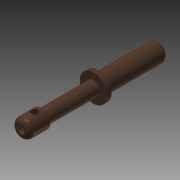
# Autodesk Inventor part: ConnectorPin
Saved by Autodesk Inventor 2014 SP2 (Build 180246200, 246)
## iProperties
Created: 2015-09-20
Part Number: ConnectorPin
Material: Generic
Document SubType Name: Modeling
Designer: Lukasz Szmit
Density: 1 g/cm^3
Appearance: Default
Mass: 0.322592 g
Surface Area: 4.28963 cm^2
Volume: 0.322592 cm^3
Author: Lukasz Szmit
Autodesk Inventor part; units mm, degrees
ref_plane "YZ Plane" through (0, 0, 0) normal (1, 0, 0) x (0, 1, 0)
ref_plane "XZ Plane" through (0, 0, 0) normal (0, 1, 0) x (-1, 0, 0)
sketch "Sketch1" plane through (0, 0, 0) normal (0, 0, 1) x (1, 0, 0)
  line L0 (-16.5001, 0.5) -> (-16.5001, -0.5)
  line L1 (-13.5001, 14) -> (-13.5001, -15.5)
  line L2 (-15.5001, 0.5) -> (-16.5001, 0.5)
  line L3 (-15.5001, 0.5) -> (-15.5001, 13)
  arc A0 (-14.5001, 14) -> (-15.5001, 13) centre (-14.5001, 13) ccw
  line L4 (-14.5001, 14) -> (-13.5001, 14)
  line L5 (-16.5001, -0.5) -> (-15.0001, -0.5)
  line L6 (-15.0001, -12) -> (-15.0001, -0.5)
  line L7 (-15.5001, -12) -> (-15.0001, -12)
  line L8 (-15.5001, -15.5318) -> (-15.5001, -12)
  line L9 (-13.5001, -15.5) -> (-14.2501, -15.5)
  arc A1 (-15.5001, -15.5318) -> (-14.2501, -16.5) centre (-14.5001, -15.5318) ccw
  line L10 (-14.2501, -15.5) -> (-14.2501, -16.5)
  dimension "d3" = 0.75
  dimension "d10" = 30.5
  dimension "d11" = 1
  dimension "d12" = 2
  dimension "d13" = 1
  dimension "d14" = 1.5
  dimension "d15" = 1
  dimension "d16" = 1.5
  dimension "d17" = 1
  dimension "d18" = 0.5
  dimension "d19" = 4.5
  dimension "d20" = 14.5
  dimension "d22" = 11.5
  dimension "d23" = 2
  dimension "d24" = 1
  constraints: 22 end point, 4 point on circle, 3 perpendicular, 3 tangent, 2 centre point, 2 parallel, 1 equal radius
  measures "d3" distance of L1.end L9.end
  measures "d10" vertical distance of L10.end L1.start
  measures "d11" distance of L0.start L0.end
  measures "d12" distance between parallel lines of L3 L1
  measures "d13" radius of A0
  measures "d14" distance between parallel lines of L6 L1
  measures "d15" distance of L2.start L0.start
  measures "d16" distance of L0.end L5.end
  measures "d17" radius of A1
  measures "d18" distance of L7.start L6.start
  measures "d19" vertical distance of L10.end L7.start
  measures "d20" vertical distance of L5.end L1.start
  measures "d22" distance of L6.start L5.end
  measures "d23" distance between parallel lines of L1 L8
  measures "d24" distance of L9.end L10.end
revolve "Revolution1" add sketch "Sketch1" angle 360 about axis through (-13.5001, 14, 0) along (0, -1, 0)
ref_plane "Work Plane1" through (-13.5001, -13.7659, 2) normal (0, 0, 1) x (1, 0, 0)
sketch "Sketch2" plane through (-13.5001, -13.7659, 2) normal (0, 0, 1) x (1, 0, 0)
  line L0 (0, -1.7659) -> (0, 1.7659) construction
  line L1 (2.2361, 13.2659) -> (-2.2361, 13.2659) construction
  line L2 (-2.2361, 13.2659) -> (-2.2361, 14.2659) construction
  line L3 (-2.2361, 14.2659) -> (0, 14.2659) construction
  line L4 (0, 14.2659) -> (0, 26.7659) construction
  line L5 (2.2361, 14.2659) -> (2.2361, 13.2659) construction
  line L6 (0, 14.2659) -> (2.2361, 14.2659) construction
  point P0 (13.5001, 13.7659)
  point P1 (0, 0.2659)
  dimension "d26" = 1.5
  constraints: 1 point on line
  measures "d26" distance of point (0, 0.266) L0.end
hole "Hole1" at (-13.5001, -13.5, 2) direction (0, 0, -1) diameter 1.5 end through all
body "Solid1"
